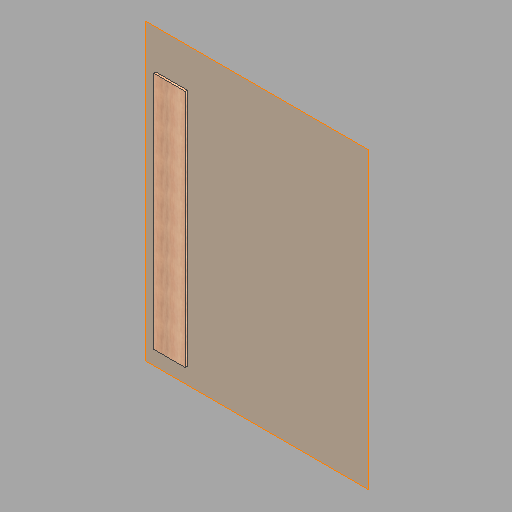
# Autodesk Inventor part: SH.1
Saved by Autodesk Inventor 2025.2 (Build 292293000, 293)
## iProperties
Created: 2025-01-27
Part Number: SH.1
Material: Wood (Birch)
Document SubType Name: Modeling
Designer: Anna
Density: 0.55 g/cm^3
Appearance: Birch - Natural Polished
Mass: 6245.93 g
Surface Area: 12841.9 cm^2
Volume: 11356.2 cm^3
Author: Anna
Autodesk Inventor part; units mm, degrees
ref_plane "YZ Plane" through (0, 0, 0) normal (1, 0, 0) x (0, 1, 0)
ref_plane "XZ Plane" through (0, 0, 0) normal (0, 1, 0) x (-1, 0, 0)
ref_plane "XY Plane" through (0, 0, 0) normal (0, 0, 1) x (1, 0, 0)
ref_plane "Work Plane3" through (0, 0, -25.4) normal (0, 0, 1) x (1, 0, 0)
sketch "Sketch1" plane through (0, 0, -25.4) normal (0, 0, 1) x (1, 0, 0)
  line L0 (-902, -1168) -> (-622.6, -1168)
  line L1 (-622.6, -1168) -> (-622.6, 965.6)
  line L2 (-622.6, 965.6) -> (-902, 965.6)
  line L3 (-902, 965.6) -> (-902, -1168)
  point P0 (0, 0)
  dimension "d0" = 279.4
  dimension "d1" = 2133.6
  constraints: 8 end point, 2 parallel, 1 horizontal, 1 perpendicular
  measures "d0" distance of L2.end L1.end
  measures "d1" distance of L1.end L0.end
extrude "Extrusion1" add sketch "Sketch1" along normal blind 19.05
body "Solid1"
